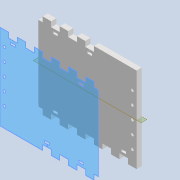
# Autodesk Inventor part: 00_Baseplate_Simmo_side2_v2
Saved by Autodesk Inventor 2022 (Build 260153000, 153)
## iProperties
Created: 2022-08-03
Part Number: 00_Baseplate_Simmo_side2_v2
Material: Generic
Document SubType Name: Modeling
Designer: wanghaoran
Density: 1 g/cm^3
Appearance: Default
Author: wanghaoran
Autodesk Inventor part; units mm, degrees
ref_plane "YZ Plane" through (0, 0, 0) normal (1, 0, 0) x (0, 1, 0)
ref_plane "XZ Plane" through (0, 0, 0) normal (0, 1, 0) x (-1, 0, 0)
ref_plane "XY Plane" through (0, 0, 0) normal (0, 0, 1) x (1, 0, 0)
sketch "Sketch1" plane through (0, 0, 0) normal (0, 0, 1) x (1, 0, 0)
  line L0 (-20, 6) -> (-10, 6) projected
  line L1 (-70, 0) -> (-70, 6) projected
  line L2 (-75, 6) -> (-70, 6) projected
  line L3 (-75, 0) -> (-75, 6) projected
  line L4 (-75, 0) -> (-70, 0) projected
  line L5 (40, -67) -> (40, -9) projected
  line L6 (40, 6) -> (-75, 6)
  line L7 (-75, 6) -> (-75, -94)
  line L8 (-75, -94) -> (40, -94)
  line L9 (40, -94) -> (40, 6)
  dimension "d85" = 115
  dimension "d86" = 100
  constraints: 8 end point, 2 parallel, 1 horizontal, 1 perpendicular, 1 point on line
  measures "d85" distance of L8.end L7.end
  measures "d86" distance of L7.end L6.end
extrude "Extrusion1" add sketch "Sketch1" along normal blind 6 contours L0 L6 L9 L5 L8 L7 L4 L1
ref_plane "Work Plane1" through (-75, -44, 0) normal (0, -1, 0) x (1, 0, 0)
sketch "Sketch2" plane through (0, 0, 6) normal (0, 0, 1) x (1, 0, 0)
  line L0 (-60, 6) -> (-60, 0) projected
  line L1 (-60, 0) -> (-50, 0) projected
  line L2 (-50, 0) -> (-50, 6) projected
  line L3 (-40, 0) -> (-30, 0) projected
  line L4 (-30, 0) -> (-30, 6) projected
  line L5 (-40, 6) -> (-40, 0) projected
  line L6 (-20, 0) -> (-10, 0) projected
  line L7 (-20, 6) -> (-20, 0) projected
  line L8 (-10, 0) -> (-10, 6) projected
  line L9 (40, 6) -> (-70, 6) projected
  line L10 (-50, 6) -> (-49.9, 6)
  line L11 (-49.9, 6) -> (-49.9, 0)
  line L12 (-49.9, 0) -> (-50, 0)
  line L13 (-50, 0) -> (-50, 6)
  line L14 (-60, 6) -> (-60.1, 6)
  line L15 (-60.1, 6) -> (-60.1, 0)
  line L16 (-60.1, 0) -> (-60, 0)
  line L17 (-60, 0) -> (-60, 6)
  point P0 (0, 0)
  dimension "d5" = 0.1
  dimension "d6" = 6
  dimension "d7" = 0.1
  dimension "d8" = 6
  constraints: 16 end point, 4 parallel, 2 horizontal, 2 perpendicular
  measures "d5" distance of L11.end L12.end
  measures "d6" distance of L10.end L11.end
  measures "d7" distance of L16.end L15.end
  measures "d8" distance of L15.end L14.end
extrude "Extrusion2" cut sketch "Sketch2" against normal blind 6 contours L9 L2 L1 L0 | L0 L16 L15 L9 | L9 L11 L12 L2
pattern_linear "Rectangular Pattern1" count 3 spacing 20 along (1, 0, 0) of "Extrusion2"
sketch "Sketch3" plane through (0, 0, 6) normal (0, 0, 1) x (1, 0, 0)
  circle A0 centre (35, -76.5) radius 1.6
  line L0 (-90, -94) -> (40, -94) projected
  line L1 (40, -94) -> (40, 6) projected
  circle A1 centre (35, -61.5) radius 1.6
  circle A2 centre (35, -46.5) radius 1.6
  circle A3 centre (35, -31.5) radius 1.6
  circle A4 centre (35, -16.5) radius 1.6
  point P0 (0, 0)
  point P1 (35, -59)
  point P2 (35, -39)
  point P3 (35, -29)
  point P4 (35, -49)
  point P5 (35, -19)
  dimension "d73" = 3.2
  dimension "d74" = 17.5
  dimension "d75" = 5
  dimension "d78" = 15
  constraints: 5 centre point, 1 vertical, 8 other
  measures "d73" diameter of A0
  measures "d74" distance from line of L0 A0.centre
  measures "d75" distance from line of L1 A0.centre
  measures "d78" distance of A0.centre A1.centre
sketch "Sketch4" plane through (0, 0, 6) normal (0, 0, 1) x (1, 0, 0)
  line L0 (-60.1, 0) -> (-60.1, 6) projected
  line L1 (-60, 0) -> (-50, 0) projected
  line L2 (-49.9, 6) -> (-49.9, 0) projected
  line L3 (-49.9, 0) -> (-60.1, 0) projected
  line L4 (66, -44) -> (-116, -44) projected
  line L5 (-60.1, -88) -> (-60.1, -94)
  line L6 (-49.9, -94) -> (-49.9, -88)
  line L7 (-49.9, -88) -> (-60.1, -88)
  line L8 (-90, -94) -> (40, -94) projected
  line L9 (-69.9, -94) -> (-69.9, -88)
  line L10 (-69.9, -88) -> (-80.1, -88)
  line L11 (-80.1, -88) -> (-80.1, -94)
  line L12 (-29.9, -94) -> (-29.9, -88)
  line L13 (-29.9, -88) -> (-40.1, -88)
  line L14 (-40.1, -88) -> (-40.1, -94)
  line L15 (-49.9, -94) -> (-49.9, -88)
  line L16 (-49.9, -88) -> (-60.1, -88)
  line L17 (-60.1, -88) -> (-60.1, -94)
  line L18 (-9.9, -94) -> (-9.9, -88)
  line L19 (-9.9, -88) -> (-20.1, -88)
  line L20 (-20.1, -88) -> (-20.1, -94)
  line L21 (-29.9, -94) -> (-29.9, -88)
  line L22 (-29.9, -88) -> (-40.1, -88)
  line L23 (-40.1, -88) -> (-40.1, -94)
  line L24 (10.1, -94) -> (10.1, -88)
  line L25 (10.1, -88) -> (-0.1, -88)
  line L26 (-0.1, -88) -> (-0.1, -94)
  line L27 (-9.9, -94) -> (-9.9, -88)
  line L28 (-9.9, -88) -> (-20.1, -88)
  line L29 (-20.1, -88) -> (-20.1, -94)
  line L30 (30.1, -94) -> (30.1, -88)
  line L31 (30.1, -88) -> (19.9, -88)
  line L32 (19.9, -88) -> (19.9, -94)
  line L33 (10.1, -94) -> (10.1, -88)
  line L34 (10.1, -88) -> (-0.1, -88)
  line L35 (-0.1, -88) -> (-0.1, -94)
  point P0 (0, 0)
  point P1 (19.9, -94)
  point P2 (30.1, -94)
  point P3 (-0.1, -94)
  point P4 (10.1, -94)
  point P5 (-20.1, -94)
  point P6 (-9.9, -94)
  point P7 (-40.1, -94)
  point P8 (-29.9, -94)
  point P9 (-80.1, -94)
  point P10 (-69.9, -94)
  dimension "d16" = 20
  dimension "d19" = 20
  constraints: 60 end point, 4 symmetric about line, 2 collinear, 2 horizontal, 61 other
  measures "d16" distance of L6.start L9.start
  measures "d19" distance of L6.start L12.start
extrude "Extrusion4" cut sketch "Sketch4" against normal blind 6
sketch "Sketch6" plane through (0, 0, 6) normal (0, 0, 1) x (1, 0, 0)
  line L0 (-69.9, -88) -> (-75, -88) projected
  line L1 (-75, -88) -> (-74.8, -88)
  line L2 (-74.8, -88) -> (-74.8, -86)
  line L3 (-74.8, -86) -> (-75, -86)
  line L4 (-75, -86) -> (-75, -88)
  line L5 (-75, -88) -> (-75.2, -88)
  line L6 (-75.2, -88) -> (-75.2, -86)
  line L7 (-75.2, -86) -> (-75, -86)
  line L8 (-75, -86) -> (-75, -88)
  point P0 (0, 0)
  point P1 (-80.1, -88)
  dimension "d40" = 0.2
  dimension "d41" = 2
  dimension "d42" = 0.2
  dimension "d43" = 2
  constraints: 17 end point, 4 parallel, 2 horizontal, 2 perpendicular
  measures "d40" distance of L3.end L2.end
  measures "d41" distance of L2.end L1.end
  measures "d42" distance of L6.end L7.end
  measures "d43" distance of L5.end L6.end
extrude "Extrusion6" cut sketch "Sketch6" against normal blind 0.2
sketch "Sketch7" plane through (0, 0, 6) normal (0, 0, 1) x (1, 0, 0)
  line L0 (27.75, -85) -> (22.25, -85)
  line L1 (22.25, -85) -> (22.25, -82.6)
  line L2 (22.25, -82.6) -> (27.75, -82.6)
  line L3 (27.75, -82.6) -> (27.75, -85)
  line L4 (10.1, -94) -> (19.9, -94) projected
  line L5 (30.1, -88) -> (30.1, -94) projected
  line L6 (-57.75, -82.6) -> (-52.25, -82.6)
  line L7 (-52.25, -82.6) -> (-52.25, -85)
  line L8 (-52.25, -85) -> (-57.75, -85)
  line L9 (-57.75, -85) -> (-57.75, -82.6)
  line L10 (-12.25, -5.4) -> (-17.75, -5.4)
  line L11 (-17.75, -5.4) -> (-17.75, -3)
  line L12 (-17.75, -3) -> (-12.25, -3)
  line L13 (-12.25, -3) -> (-12.25, -5.4)
  line L14 (-20.1, 6) -> (-29.9, 6) projected
  line L15 (-9.9, 6) -> (-9.9, 0) projected
  line L16 (-52.25, -5.4) -> (-57.75, -5.4)
  line L17 (-57.75, -3) -> (-52.25, -3)
  line L18 (-52.25, -3) -> (-52.25, -5.4)
  line L19 (-57.75, -5.4) -> (-57.75, -3)
  point P0 (0, 0)
  dimension "d4" = 0
  dimension "d49" = 5.5
  dimension "d50" = 2.4
  dimension "d51" = 9
  dimension "d52" = 2.35
  dimension "d55" = 80
  dimension "d60" = 5.5
  dimension "d61" = 2.4
  dimension "d62" = 9
  dimension "d63" = 2.35
  dimension "d66" = 40
  constraints: 32 end point, 4 horizontal, 4 parallel, 2 collinear, 2 perpendicular, 14 other
  measures "d49" distance of L1.end L2.end
  measures "d50" distance of L0.end L1.end
  measures "d51" distance between parallel lines of L4 L0
  measures "d52" distance between parallel lines of L5 L3
  measures "d55" distance of L1.end L6.start
  measures "d60" distance of L11.end L12.end
  measures "d61" distance of L10.end L11.end
  measures "d62" distance between parallel lines of L14 L12
  measures "d63" distance between parallel lines of L15 L13
  measures "d66" distance of L10.start L16.start
extrude "Extrusion7" cut sketch "Sketch7" against normal blind 6
extrude "Extrusion8" cut sketch "Sketch3" against normal through all
body "Solid1"
